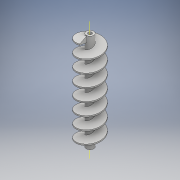
# Autodesk Inventor part: Axis
Saved by Autodesk Inventor 2017 (Build 210142000, 142)
## iProperties
Created: 2016-05-10
Part Number: Axis
Material: Generic
Document SubType Name: Modeling
Designer: Bastli
Density: 1 g/cm^3
Appearance: Default
Author: Bastli
Autodesk Inventor part; units mm, degrees
ref_plane "YZ Plane" through (0, 0, 0) normal (1, 0, 0) x (0, 1, 0)
ref_plane "XZ Plane" through (0, 0, 0) normal (0, 1, 0) x (-1, 0, 0)
ref_plane "XY Plane" through (0, 0, 0) normal (0, 0, 1) x (1, 0, 0)
sketch "Sketch1" plane through (0, 0, 0) normal (0, 0, 1) x (1, 0, 0)
  circle A0 centre (0, 0) radius 3
  dimension "Axis_diameter" = 6
  constraints: 1 centre point, 1 coincident
  measures "Axis_diameter" diameter of A0
extrude "Axis" add sketch "Sketch1" along normal blind 80
sketch "CoilSketch" plane through (0, 0, 0) normal (1, 0, 0) x (0, 1, 0)
  line L0 (3, 0) -> (10, 1.8756)
  line L1 (10, 1.8756) -> (10, 2.8756)
  line L2 (10, 2.8756) -> (3, 4.7513)
  line L3 (3, 0) -> (9.25, 0) construction
  line L4 (3, 4.7513) -> (8, 4.7513) construction
  line L5 (3, 0) -> (3, 80) projected
  line L6 (3, 4.7513) -> (3, 0)
  point P0 (0, 0)
  dimension "Lower_Pitch" = 15
  dimension "Upper_Width" = 1
  dimension "Height" = 7
  dimension "Upper_Pitch" = 15
  dimension "Base_Width" = 4.7513
  constraints: 12 end point, 2 horizontal, 1 equal length, 1 perpendicular
  measures "Lower_Pitch" angle of L3 L0
  measures "Upper_Width" distance of L0.end L1.end
  measures "Height" horizontal distance of L0.start L0.end
  measures "Upper_Pitch" angle of L4 L2
  measures "Base_Width" distance of L0.start L2.end
coil "Coil1" sketch "CoilSketch" operation add axis through (0, 0, -10) along (0, 0, 1) pitch 10 turns 7.524871 hand right
sketch "Sketch3" plane through (0, 0, 80) normal (0, 0, 1) x (1, 0, 0)
  circle A0 centre (0, 0) radius 1.5
  dimension "Hole_Diameter" = 3
  constraints: 1 centre point, 1 coincident
  measures "Hole_Diameter" diameter of A0
extrude "Extrusion2" cut sketch "Sketch3" against normal blind 5
equation "\"Height\" = -0.5 * Axis_diameter + 0.5 * Total_Diameter"
equation "\"d8\" = Axis_length - Base_Width"
equation "\"Total_Diameter\" = 20"
equation "\"Axis_length\" = 80"
body "Solid1"
